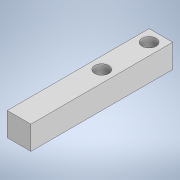
# Autodesk Inventor part: アーム10×10×60
Saved by Autodesk Inventor 2021 (Build 250183000, 183)
## iProperties
Created: 2021-10-09
Part Number: アーム10×10×60
Material: 一般
Document SubType Name: Modeling
Designer: ryusei
Density: 1 g/cm^3
Appearance: 既定
Author: ryusei
Autodesk Inventor part; units mm, degrees
ref_plane "YZ Plane" through (0, 0, 0) normal (1, 0, 0) x (0, 1, 0)
ref_plane "XZ Plane" through (0, 0, 0) normal (0, 1, 0) x (-1, 0, 0)
ref_plane "XY Plane" through (0, 0, 0) normal (0, 0, 1) x (1, 0, 0)
sketch "スケッチ1" plane through (0, 0, 0) normal (0, 0, 1) x (1, 0, 0)
  line L0 (0, 0) -> (10, 0)
  line L1 (10, 0) -> (10, 10)
  line L2 (10, 10) -> (0, 10)
  line L3 (0, 10) -> (0, 0)
  dimension "d0" = 10
  dimension "d1" = 10
  constraints: 8 end point, 2 parallel, 1 horizontal, 1 perpendicular
  measures "d0" distance of L0.end L1.end
  measures "d1" distance of L1.end L2.end
extrude "押し出し1" add sketch "スケッチ1" along normal blind 60
sketch "スケッチ2" plane through (0, 10, 0) normal (0, 1, 0) x (1, 0, 0)
  line L0 (0, 0) -> (0, -60) projected
  line L1 (10, 0) -> (0, 0) projected
  point P0 (5, -5)
  dimension "d4" = 5
  dimension "d5" = 5
  measures "d4" distance from line of L0 point (5, -5)
  measures "d5" distance from line of L1 point (5, -5)
hole "穴1" at (5, 10, 5) direction (0, -1, 0) diameter 6 end through all
sketch "スケッチ3" plane through (0, 10, 0) normal (0, 1, 0) x (1, 0, 0)
  line L0 (0, 0) -> (0, -60) projected
  line L1 (10, 0) -> (0, 0) projected
  point P0 (5, -25)
  dimension "d13" = 5
  dimension "d14" = 25
  measures "d13" distance from line of L0 point (5, -25)
  measures "d14" distance from line of L1 point (5, -25)
hole "穴2" at (5, 10, 25) direction (0, -1, 0) diameter 6 end through all
